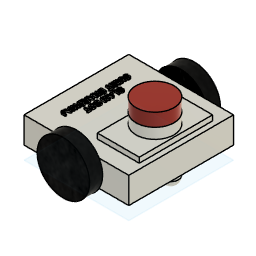
myrobot v2 (Autodesk Fusion 360 design; units mm, degrees)
Autodesk Fusion 360 part; units mm, degrees
sketch "Sketch1" plane through (0, 0, 0) normal (0, 0, 1) x (1, 0, 0)
  line L0 (100, 100) -> (-100, 100)
  line L1 (-100, 100) -> (-100, -100)
  line L2 (-100, -100) -> (100, -100)
  line L3 (100, -100) -> (100, 100)
  constraint horizontal L0
  constraint vertical L1
  constraint horizontal L2
  constraint vertical L3
extrude "Extrude1" add sketch "Sketch1" along normal blind 50 makes body 1
sketch "Sketch2" plane through (0, 0, 0) normal (0, 0, -1) x (1, 0, 0)
  line L0 (100, -100) -> (100, 100)
  line L1 (100, 100) -> (-100, 100)
  line L2 (-100, 100) -> (-100, -100)
  line L3 (-100, -100) -> (100, -100)
sketch "Sketch3" plane through (0, -100, 0) normal (0, -1, 0) x (1, 0, 0)
  line L0 (-100, 0) -> (100, 0)
  line L1 (100, 0) -> (100, 50)
  line L2 (100, 50) -> (-100, 50)
  line L3 (-100, 50) -> (-100, 0)
  circle A0 centre (0, 25) radius 50
extrude "Extrude2" add sketch "Sketch3" along normal blind 25 separate body contours L0 L2 A0 | L0 A0 | L2 A0 makes body 2
mirror "Mirror1" about plane through (0, 0, 0) normal (0, 1, 0) of bodies 2 makes body 3
ref_plane "WorkPlane1" through (0, -116.0104, -25) normal (0, 0, -1) x (-1, 0, 0)
move_body "Move1" bodies 1 2 3 to x (1, 0, 0) y (0, 1, 0) z (0, 0, 1) at (0, 0, 25)
sketch "Sketch4" plane through (0, 0, 0) normal (0, 0, 1) x (1, 0, 0)
  circle A0 centre (-80, 0) radius 15
  circle A1 centre (80, 0) radius 15
extrude "Extrude3" add sketch "Sketch4" along normal blind 25 bodies 1
fillet "Fillet1" radius 15 1 edges at (-93.9849, -5.4242, 0) on bodies 1
fillet "Fillet2" radius 15 1 faces at (74.7811, 1.9491, 0) on bodies 1
sketch "Sketch5" plane through (0, 0, 75) normal (0, 0, 1) x (-1, 0, 0)
  line L0 (-100, 100) -> (-100, -100)
  line L1 (-100, -100) -> (100, -100)
  line L2 (100, -100) -> (100, 100)
  line L3 (100, 100) -> (-100, 100)
  line L4 (-90, -70) -> (-10, -70)
  line L5 (-10, -70) -> (-10, 70)
  line L6 (-10, 70) -> (-90, 70)
  line L7 (-90, 70) -> (-90, -70)
  constraint horizontal L4
  constraint vertical L5
  constraint horizontal L6
  constraint vertical L7
extrude "Extrude4" add sketch "Sketch5" along normal blind 10 contours L4 L5 L6 L7 bodies 1
sketch "Sketch6" plane through (0, 0, 85) normal (0, 0, 1) x (-1, 0, 0)
  line L0 (-90, 70) -> (-90, -70)
  line L1 (-90, -70) -> (-10, -70)
  line L2 (-10, -70) -> (-10, 70)
  line L3 (-10, 70) -> (-90, 70)
  circle A0 centre (-50, 0) radius 36.2774
extrude "Extrude5" add sketch "Sketch6" along normal blind 20 contours A0 bodies 1
extrude "Extrude6" add 1 faces at (61.2971, -7.0087, 105) along direction (0, 0, 1) blind 25 separate body on bodies 1 makes body 4
sketch "Sketch7" plane through (-100, 0, 0) normal (-1, 0, 0) x (0, -1, 0)
  line L0 (-100, 25) -> (100, 25)
  line L1 (100, 25) -> (100, 75)
  line L2 (100, 75) -> (-100, 75)
  line L3 (-100, 75) -> (-100, 25)
  line L4 (-80, 30) -> (80, 30) construction
  line L5 (80, 30) -> (80, 70) construction
  line L6 (80, 70) -> (-80, 70) construction
  line L7 (-80, 70) -> (-80, 30) construction
  dimension "d20" = 10
  text T0 "SLAM BOT\nSUMIT BHARDWAJ" font "Arial" height 10 bold align centre middle in box 160 x 40 at (-80, 30) x (1, 0) y (0, 1) spacing 1 kerned
extrude "Extrude7" add sketch "Sketch7" along normal blind 3 text T0 bodies 1
sketch "Sketch8" plane through (0, 0, 75) normal (0, 0, 1) x (-1, 0, 0)
  line L0 (-90, 70) -> (-10, 70)
  line L1 (-10, 70) -> (-10, -70)
  line L2 (-10, -70) -> (-90, -70)
  line L3 (-90, -70) -> (-90, 70)
  line L4 (-100, 100) -> (-100, -100)
  line L5 (-100, -100) -> (100, -100)
  line L6 (100, -100) -> (100, 100)
  line L7 (100, 100) -> (-100, 100)
  line L8 (80, -80) -> (80, 80) construction
  line L9 (80, 80) -> (30, 80) construction
  line L10 (30, 80) -> (30, -80) construction
  line L11 (30, -80) -> (80, -80) construction
  dimension "d23" = 10
  text T0 "SLAM BOT\nSUMIT BHARDWAJ" font "Arial" height 10 bold align centre middle in box 160 x 50 at (80, -80) x (0, 1) y (-1, 0) spacing 1 kerned
extrude "Extrude8" add sketch "Sketch8" along normal blind 3 text T0 bodies 1
copy_body "Body->Comp1" bodies 1 removing the originals makes body 5 in component "base_link"
copy_body "Body->Comp2" bodies 2 removing the originals makes body 6 in component "right_wheel"
copy_body "Body->Comp3" bodies 3 removing the originals makes body 7 in component "left_wheel"
copy_body "Body->Comp4" bodies 4 removing the originals makes body 8 in component "lidar"
component "base_link" placed x (1, 0, 0) y (0, 1, 0) z (0, 0, 1) at (0, 0, 0)
component "right_wheel" placed x (1, 0, 0) y (0, 1, 0) z (0, 0, 1) at (0, 0, 0)
component "left_wheel" placed x (1, 0, 0) y (0, 1, 0) z (0, 0, 1) at (0, 0, 0)
component "lidar" placed x (1, 0, 0) y (0, 1, 0) z (0, 0, 1) at (0, 0, 0)
named bodies: "base_link", "right_wheel", "left_wheel", "lidar"
